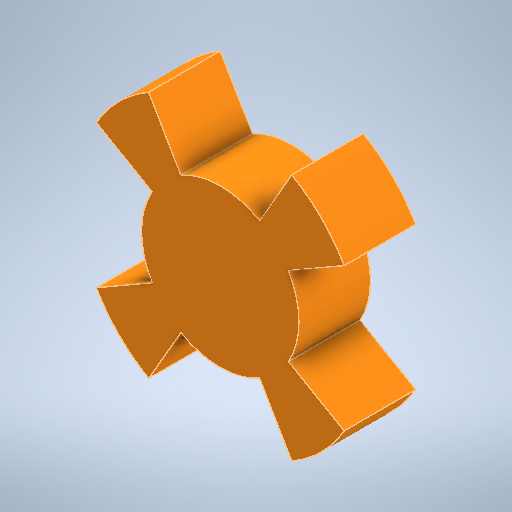
# Autodesk Inventor part: NYLON-JAW
Saved by Autodesk Inventor 2025.3 (Build 293356030, 356C)
## iProperties
Created: 2025-10-06
Part Number: NYLON-JAW
Material: Generic
Document SubType Name: Modeling
Designer: lstk1ng
Density: 1 g/cm^3
Appearance: Orange
Author: lstk1ng
Autodesk Inventor part; units mm, degrees
ref_plane "YZ Plane" through (0, 0, 0) normal (1, 0, 0) x (0, 1, 0)
ref_plane "XZ Plane" through (0, 0, 0) normal (0, 1, 0) x (-1, 0, 0)
ref_plane "XY Plane" through (0, 0, 0) normal (0, 0, 1) x (1, 0, 0)
sketch "Sketch1" plane through (0, 0, 0) normal (0, 0, 1) x (1, 0, 0)
  line L0 (-9.5263, 5.5) -> (-17.3205, 10)
  line L1 (0, 0) -> (20, 0) construction
  line L2 (-9.5263, -5.5) -> (-17.3205, -10)
  line L3 (0, 0) -> (20, 0) construction
  line L4 (5.5, 9.5263) -> (10, 17.3205)
  line L5 (0, 0) -> (20, 0) construction
  line L6 (-5.5, 9.5263) -> (-10, 17.3205)
  line L7 (0, 0) -> (20, 0) construction
  line L8 (5.5, -9.5263) -> (10, -17.3205)
  line L9 (-5.5, -9.5263) -> (-10, -17.3205)
  line L10 (0, 0) -> (0, 20) construction
  line L11 (9.5263, 5.5) -> (17.3205, 10)
  line L12 (9.5263, -5.5) -> (17.3205, -10)
  arc A0 (17.3205, 10) -> (10, 17.3205) centre (0, 0) ccw
  arc A1 (-10, 17.3205) -> (-17.3205, 10) centre (0, 0) ccw
  arc A2 (-17.3205, -10) -> (-10, -17.3205) centre (0, 0) ccw
  arc A3 (10, -17.3205) -> (17.3205, -10) centre (0, 0) ccw
  arc A4 (-9.5263, 5.5) -> (-9.5263, -5.5) centre (0, 0) ccw
  arc A5 (5.5, 9.5263) -> (-5.5, 9.5263) centre (0, 0) ccw
  arc A6 (-5.5, -9.5263) -> (5.5, -9.5263) centre (0, 0) ccw
  arc A7 (9.5263, -5.5) -> (9.5263, 5.5) centre (0, 0) ccw
  dimension "d2" = 150
  dimension "d3" = 150
  dimension "d4" = 60
  dimension "d5" = 120
  constraints: 26 end point, 16 point on circle, 8 centre point, 4 horizontal, 4 symmetric about line, 2 coincident, 1 vertical
  measures "d2" angle of L1 L0
  measures "d3" angle of L2 L3
  measures "d4" angle of L5 L4
  measures "d5" angle of L7 L6
extrude "Extrusion1" add sketch "Sketch1" along normal blind 10
body "Solid1"
